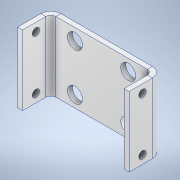
# Autodesk Inventor part: servo_bracket
Saved by Autodesk Inventor 2020 (Build 240168000, 168)
## iProperties
Created: 2020-06-27
Part Number: servo_bracket
Material: アルミニウム 6061
Document SubType Name: Sheet Metal
Designer: haya
Density: 2.7 g/cm^3
Sheet Metal Rule: Default_mm
Appearance: アルミニウム - フラット
Author: haya
Autodesk Inventor part; units mm, degrees
ref_plane "YZ Plane" through (0, 0, 0) normal (1, 0, 0) x (0, 1, 0)
ref_plane "XZ Plane" through (0, 0, 0) normal (0, 1, 0) x (-1, 0, 0)
ref_plane "XY Plane" through (0, 0, 0) normal (0, 0, 1) x (1, 0, 0)
sketch "スケッチ1" plane through (0, 0, 0) normal (0, 0, 1) x (1, 0, 0)
  line L0 (0, 0) -> (30.5, 0)
  line L1 (30.5, 0) -> (30.5, 21)
  line L2 (30.5, 21) -> (0, 21)
  line L3 (0, 21) -> (0, 0)
  dimension "d0" = 30.5
  dimension "d1" = 21
  measures "d0" distance of L0.start L0.end
  measures "d1" distance of L2.end L0.start
extrude "プレート1" add sketch "スケッチ1" along normal blind 1.5
sketch "スケッチ2" plane through (30.5, 21, 1.5) normal (1, 0, 0) x (0, 1, 0)
  line L0 (-21, 0) -> (0, 0)
  line L1 (0, 0) -> (0, 8.5)
  line L2 (0, 8.5) -> (-21, 8.5)
  line L3 (-21, 8.5) -> (-21, 0)
  constraints: 6 end point, 1 horizontal, 1 perpendicular, 1 vertical
edge flange "フランジ1" height 10 angle 90 thickness 1.5 bend radius 1.5 thickness toward (1, 0, 0) relief tear relief width 1.5 relief depth 0.75 corner gap 1.5 corner form 0 edges at (30.5, 10.5, 1.5) (0, 10.5, 1.5) wall of the first edge with corners at (30.5, 0, 1.5) (30.5, 21, 1.5) (30.5, 21, 10) (30.5, 0, 10)
bend "曲げ1"
corner "コーナー1"
sketch "スケッチ3" plane through (32, 0, 10) normal (1, 0, 0) x (0, 0, -1)
  line L0 (4, 0) -> (4, 21) construction
  line L1 (7, 21) -> (0, 21) projected
  line L2 (0, 21) -> (0, 0) projected
  line L3 (0, 10.5) -> (4, 10.5)
  point P0 (10, 0)
  point P1 (4, 2.5)
  point P2 (4, 18.5)
  dimension "d15" = 4
  dimension "d16" = 16
  constraints: 4 end point, 2 midpoint, 2 point on line, 1 horizontal, 1 symmetric about line, 1 vertical
  measures "d15" distance between parallel lines of L0 L2
  measures "d16" distance of point (4, 18.5) point (4, 2.5)
hole "穴1" at (32, 2.5, 6) at (32, 18.5, 6) direction (-1, 0, 0) diameter 2.2 end through all
sketch "スケッチ4" plane through (0, 0, 0) normal (0, 0, -1) x (-1, 0, 0)
  line L0 (-32, 0) -> (-32, 21) projected
  line L1 (-32, 10.5) -> (1.5, 10.5)
  line L2 (1.5, 21) -> (1.5, 0) projected
  line L3 (-29, 0) -> (-1.5, 0) projected
  line L4 (-15.25, 0) -> (-15.25, 21)
  line L5 (-1.5, 21) -> (-29, 21) projected
  point P0 (0, 0)
  point P1 (-23.25, 3.5)
  point P2 (-23.25, 17.5)
  point P3 (-7.25, 3.5)
  point P4 (-7.25, 17.5)
  dimension "d31" = 14
  dimension "d32" = 16
  constraints: 4 end point, 4 midpoint, 3 symmetric about line
  measures "d31" distance of point (-23.25, 17.5) point (-23.25, 3.5)
  measures "d32" distance of point (-7.25, 3.5) point (-23.25, 3.5)
hole "穴2" at (23.25, 3.5, 0) at (23.25, 17.5, 0) at (7.25, 3.5, 0) at (7.25, 17.5, 0) direction (0, 0, 1) diameter 4.5 end through all
equation "\"d22\" = Thickness"
equation "\"d29\" = Thickness"
equation "\"d2\" = Thickness"
equation "\"d3\" = BendReliefWidth"
equation "\"d4\" = BendReliefDepth"
equation "\"d5\" = MinimumRemnant"
equation "\"d6\" = TransitionRadius"
equation "\"d9\" = BendRadius"
equation "\"d10\" = CornerReliefSize"
equation "\"d11\" = GapSize"
equation "\"d12\" = JacobiRadiusSize"
equation "\"BendRadius\" = Thickness"
equation "\"BendReliefWidth\" = Thickness"
equation "\"BendReliefDepth\" = 0.5 * Thickness"
equation "\"CornerReliefSize\" = 4 * Thickness"
equation "\"MinimumRemnant\" = 2 * Thickness"
equation "\"TransitionRadius\" = BendRadius"
equation "\"JacobiRadiusSize\" = BendRadius"
equation "\"GapSize\" = Thickness"
equation "\"Thickness\" = 1.5"
